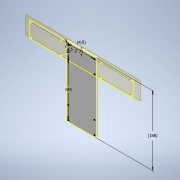
# Autodesk Inventor part: upper-lower form connector
Saved by Autodesk Inventor 2021 (Build 250183000, 183)
## iProperties
Created: 2021-11-20
Part Number: upper-lower form connector
Material: Generic
Document SubType Name: Modeling
Designer: techv
Density: 1 g/cm^3
Appearance: Default
Author: techv
Autodesk Inventor part; units mm, degrees
ref_plane "YZ Plane" through (0, 0, 0) normal (1, 0, 0) x (0, 1, 0)
ref_plane "XZ Plane" through (0, 0, 0) normal (0, 1, 0) x (-1, 0, 0)
ref_plane "Work Plane1" through (0, 0, 0) normal (0, 0, 1) x (1, 0, 0)
sketch "Sketch1" plane through (0, 0, 0) normal (0, 0, 1) x (1, 0, 0)
  arc A0 (-290.5, 45) -> (-292.5, 43) centre (-290.5, 43) ccw projected
  line L0 (-292.5, 1) -> (-292.5, 43) projected
  line L1 (-10, 1) -> (-292.5, 1) projected
  line L2 (-10, 1) -> (-10, 43) projected
  arc A1 (-10, 43) -> (-12, 45) centre (-12, 43) ccw projected
  line L3 (-12, 45) -> (-290.5, 45) projected
  circle A2 centre (-205.5, 4.5) radius 1.4 projected
  circle A3 centre (-288.25, 40.5) radius 1.4 projected
  circle A4 centre (-288.25, 4.5) radius 1.4 projected
  circle A5 centre (-97, 40.5) radius 1.4 projected
  circle A6 centre (-97, 4.5) radius 1.4 projected
  circle A7 centre (-14.25, 40.5) radius 1.4 projected
  circle A8 centre (-14.25, 4.5) radius 1.4 projected
  circle A9 centre (-205.5, 40.5) radius 1.4 projected
  line L4 (-292.5, 22) -> (-10, 22) construction
  line L5 (-151.25, 45) -> (-151.25, 1) construction
  line L6 (-191.25, 45) -> (-111.25, 45)
  line L7 (-111.25, 45) -> (-111.25, -1)
  line L8 (-111.25, -1) -> (-191.25, -1)
  line L9 (-191.25, -1) -> (-191.25, 45)
  line L10 (-191.25, 45) -> (-111.25, -1) construction
  line L11 (-111.25, 45) -> (-191.25, -1) construction
  point P0 (0, 0)
  point P1 (-151.25, 22)
  point P2 (-191.25, 1)
  point P3 (-111.25, 1)
  dimension "d0" = 80
  dimension "d1" = 46
  constraints: 16 end point, 7 midpoint, 2 parallel, 1 horizontal, 1 perpendicular, 1 point on line
  measures "d0" distance of L7.end L8.end
  measures "d1" distance of L6.end L7.end
extrude "Extrusion1" add sketch "Sketch1" along normal blind 5 contours L3 L7 L1 L9
sketch "Sketch2" plane through (-191.25, 1, 0) normal (0, -1, 0) x (1, 0, 0)
  line L0 (0, 0) -> (80, 0) projected
  line L1 (80, 0) -> (80, 5) projected
  line L2 (0, 5) -> (80, 5) projected
  line L3 (0, 0) -> (0, 5) projected
  point P0 (191.25, 0)
ref_plane "Work Plane2" through (-292.5, -143, -256) normal (0, -1, 0) x (1, 0, 0)
extrude "Extrusion2" add sketch "Sketch2" along normal up to surface (144 mm away)
sketch "Sketch3" plane through (0, 0, 5) normal (0, 0, 1) x (1, 0, 0)
  arc A0 (-290.5, 45) -> (-292.5, 43) centre (-290.5, 43) ccw projected
  line L0 (-292.5, 1) -> (-292.5, 43) projected
  line L1 (-10, 1) -> (-292.5, 1) projected
  line L2 (-10, 1) -> (-10, 43) projected
  arc A1 (-10, 43) -> (-12, 45) centre (-12, 43) ccw projected
  line L3 (-12, 45) -> (-290.5, 45) projected
  circle A2 centre (-205.5, 4.5) radius 1.4 projected
  circle A3 centre (-288.25, 40.5) radius 1.4 projected
  circle A4 centre (-288.25, 4.5) radius 1.4 projected
  circle A5 centre (-97, 40.5) radius 1.4 projected
  circle A6 centre (-97, 4.5) radius 1.4 projected
  circle A7 centre (-14.25, 40.5) radius 1.4 projected
  circle A8 centre (-14.25, 4.5) radius 1.4 projected
  circle A9 centre (-205.5, 40.5) radius 1.4 projected
  line L4 (-111.25, 45) -> (-111.25, -143) projected
  line L5 (-111.25, 45) -> (-191.25, 45) projected
  line L6 (-191.25, 45) -> (-191.25, -143) projected
  line L7 (-191.25, -143) -> (-111.25, -143) projected
  line L8 (-288.25, 40.5) -> (-14.25, 40.5) construction
  line L9 (-111.25, 45) -> (-191.25, 45) construction
  line L10 (-186.75, 45) -> (-186.75, 1) construction
  circle A10 centre (-186.75, 40.5) radius 1.5
  circle A11 centre (-115.75, 40.5) radius 1.5
  circle A12 centre (-186.75, 4.5) radius 1.5
  circle A13 centre (-115.75, 4.5) radius 1.5
  circle A14 centre (-186.75, -138.5) radius 1.5
  circle A15 centre (-115.75, -138.5) radius 1.5
  circle A16 centre (-115.75, -102.5) radius 1.5
  circle A17 centre (-186.75, -102.5) radius 1.5
  point P0 (0, 0)
  dimension "d6" = 4.5
  dimension "d7" = 4.5
  dimension "d8" = 3
  dimension "d11" = 71
  dimension "d14" = 36
  dimension "d17" = 188
  dimension "d20" = 143
  constraints: 8 centre point, 4 end point, 4 point on line, 2 vertical, 1 horizontal, 1 parallel, 1 perpendicular, 14 other
  measures "d6" distance between parallel lines of L8 L5
  measures "d7" distance between parallel lines of L10 L6
  measures "d8" diameter of A10
  measures "d11" distance of A10.centre A11.centre
  measures "d14" distance of A10.centre A12.centre
  measures "d17" distance between parallel lines of L7 L5
  measures "d20" distance of A12.centre A14.centre
extrude "Extrusion3" cut sketch "Sketch3" against normal through all contours A10 | A11 | A12 | A13 | A14 | A15 | A16 | A17
body "Solid1"
